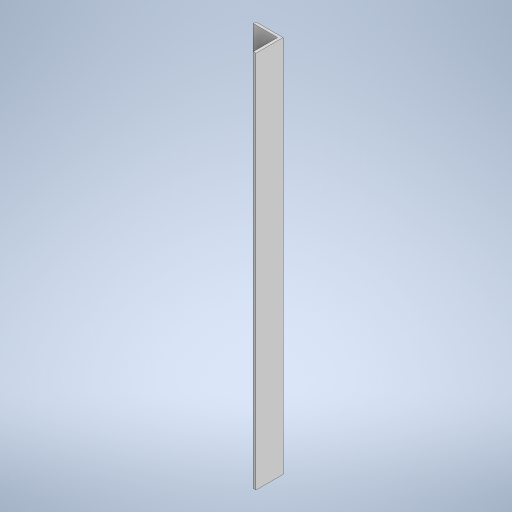
# Autodesk Inventor part: YaxisUgolok
Saved by Autodesk Inventor 2024 (Build 280153000, 153)
## iProperties
Created: 2023-06-19
Part Number: YaxisUgolok
Material: Generic
Document SubType Name: Modeling
Designer: KirikDK
Density: 1 g/cm^3
Appearance: Default
Author: KirikDK
Autodesk Inventor part; units mm, degrees
ref_plane "YZ Plane" through (0, 0, 0) normal (1, 0, 0) x (0, 1, 0)
ref_plane "XZ Plane" through (0, 0, 0) normal (0, 1, 0) x (-1, 0, 0)
ref_plane "XY Plane" through (0, 0, 0) normal (0, 0, 1) x (1, 0, 0)
sketch "Sketch1" plane through (0, 0, 0) normal (0, 1, 0) x (-1, 0, 0)
  line L0 (0, 50) -> (0, 0)
  line L1 (0, 0) -> (50, 0)
  line L2 (50, 0) -> (50, 5)
  line L3 (50, 5) -> (5, 5)
  line L4 (5, 5) -> (5, 50)
  line L5 (5, 50) -> (0, 50)
  dimension "d0" = 50
  dimension "d1" = 50
  dimension "d3" = 5
  dimension "d4" = 5
  constraints: 12 end point, 2 perpendicular, 1 vertical
  measures "d0" distance of L0.start L0.end
  measures "d1" distance of L0.end L1.end
  measures "d3" distance between parallel lines of L1 L3
  measures "d4" distance between parallel lines of L4 L0
extrude "Extrusion1" add sketch "Sketch1" along normal blind 700
body "Solid1"
